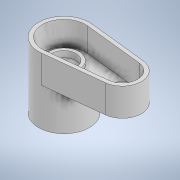
# Autodesk Inventor part: Klapphülle
Saved by Autodesk Inventor 2021 (Build 250183000, 183)
## iProperties
Created: 2021-01-08
Part Number: Klapphülle
Material: Generisch
Document SubType Name: Modeling
Designer: Jaro Machnow
Density: 1 g/cm^3
Appearance: Vorgabe
Author: Jaro Machnow
Autodesk Inventor part; units mm, degrees
ref_plane "YZ Plane" through (0, 0, 0) normal (1, 0, 0) x (0, 1, 0)
ref_plane "XZ Plane" through (0, 0, 0) normal (0, 1, 0) x (-1, 0, 0)
ref_plane "XY Plane" through (0, 0, 0) normal (0, 0, 1) x (1, 0, 0)
sketch "Skizze1" plane through (0, 0, 0) normal (0, 1, 0) x (-1, 0, 0)
  arc A0 (-2.173913, -19.881502) -> (-2.173913, 19.881502) centre (0, 0) ccw
  arc A1 (-47.630435, 14.911126) -> (-47.630435, -14.911126) centre (-46, 0) ccw
  line L0 (-2.173913, 19.881502) -> (-47.630435, 14.911126)
  line L1 (-2.173913, -19.881502) -> (-47.630435, -14.911126)
  line L2 (45.02348, 0) -> (-115.148005, 0) construction
  dimension "Klapp_d_oben" = 40
  dimension "Klapp_d_unten" = 30
  dimension "Klapp_Abstand_oben_unten" = 46
  constraints: 6 end point, 4 point on circle, 4 tangent, 2 centre point, 2 horizontal, 1 coincident, 1 point on line
  measures "Klapp_d_oben" diameter of A0
  measures "Klapp_d_unten" diameter of A1
  measures "Klapp_Abstand_oben_unten" distance of A1.centre point (0, 0)
extrude "Extrusion1" add sketch "Skizze1" along normal blind 22
sketch "Skizze2" plane through (0, 22, 0) normal (0, 1, 0) x (1, 0, 0)
  arc A0 (47.630435, -14.911126) -> (47.630435, 14.911126) centre (46, 0) ccw
  line L0 (2.173913, -19.881502) -> (47.630435, -14.911126)
  arc A1 (47.630435, -14.911126) -> (47.630435, 14.911126) centre (46, 0) ccw
  line L1 (47.630435, 14.911126) -> (2.173913, 19.881502)
  arc A2 (2.173913, 19.881502) -> (2.173913, -19.881502) centre (0, 0) ccw
  circle A3 centre (46, 0) radius 5
  dimension "Klapp_Welle_Rad_d" = 10
  constraints: 1 centre point, 1 coincident
  measures "Klapp_Welle_Rad_d" diameter of A3
extrude "Extrusion2" [suppressed]
sketch "Skizze3" plane through (0, 0, 0) normal (0, -1, 0) x (1, 0, 0)
  circle A0 centre (0, 0) radius 9.5
  dimension "Klapp_Welle_Karosserie_d" = 19
  constraints: 1 centre point, 1 coincident
  measures "Klapp_Welle_Karosserie_d" diameter of A0
extrude "Extrusion3" [suppressed]
shell "Wandung1" thickness 3 removed faces 1 at (17.326087, 22, -4.970375)
sketch "Skizze7" plane through (0, 3, 0) normal (0, 1, 0) x (1, 0, 0)
  point P0 (0, 0)
sketch "Skizze9" plane through (0, 3, 0) normal (0, 1, 0) x (1, 0, 0)
  circle A0 centre (0, 0) radius 9.5
  circle A1 centre (0, 0) radius 12
  dimension "d25" = 19
  dimension "d26" = 24
  constraints: 2 centre point, 2 coincident
  measures "d25" diameter of A0
  measures "d26" diameter of A1
extrude "Extrusion6" add sketch "Skizze9" along normal blind 3
sketch "Skizze10" plane through (0, 3, 0) normal (0, 1, 0) x (1, 0, 0)
  circle A0 centre (0, 0) radius 9.5
  constraints: 1 centre point, 1 coincident
extrude "Extrusion7" cut sketch "Skizze10" against normal blind 2
sketch "Skizze11" plane through (0, 3, 0) normal (0, 1, 0) x (1, 0, 0)
  point P0 (0, 0)
sketch "Skizze12" plane through (0, 3, 0) normal (0, 1, 0) x (1, 0, 0)
  arc A0 (47.304348, -11.928901) -> (47.304348, 11.928901) centre (46, 0) ccw
  circle A1 centre (46, 0) radius 9.5
  circle A2 centre (46, 0) radius 12
  point P0 (0, 0)
  point P1 (47.304348, -11.928901)
  dimension "d31" = 19
  constraints: 2 centre point, 2 coincident, 1 concentric
  measures "d31" diameter of A1
extrude "Extrusion8" add sketch "Skizze12" along normal blind 3
sketch "Skizze13" plane through (46, 3, 0) normal (0, 1, 0) x (1, 0, 0)
  circle A0 centre (0, 0) radius 9.5
  point P0 (-46, 0)
  constraints: 1 centre point
extrude "Extrusion9" cut sketch "Skizze13" against normal blind 2
hole "Bohrung2" at (0, 3, 0) direction (0, -1, 0) diameter 11 end through all
sketch "Skizze15" plane through (0, 0, 0) normal (0, -1, 0) x (1, 0, 0)
  circle A0 centre (0, 0) radius 20
  circle A1 centre (0, 0) radius 12.5
  dimension "d44" = 25
  constraints: 2 centre point, 2 coincident
  measures "d44" diameter of A1
extrude "Extrusion10" add sketch "Skizze15" along normal blind 30
